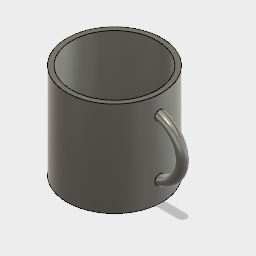
水杯 (Autodesk Fusion 360 design; units mm, degrees)
Autodesk Fusion 360 part; units mm, degrees
cylinder "圆柱体基本要素2" add diameter 20 height 20 placed x (1, 0, 0) y (0, 0, -1) z (0, 1, 0) at (0, 0, 0) makes body 1
cylinder "圆柱体基本要素3" add diameter 18 height 20 placed x (1, 0, 0) y (0, 0, -1) z (0, 1, 0) at (30, 0, 0) separate body makes body 2
torus "圆环体基本要素1" add centre line diameter 12 section diameter 2 placed x (1, 0, 0) y (0, 0, -1) z (0, 1, 0) at (65, 0, 0) separate body makes body 3
move_body "MoveFace1" bodies 3 to x (1, 0, 0) y (0, 0.173648, 0.984808) z (0, -0.984808, 0.173648) at (-80.5059, 25.9211, 54.5848) on bodies 3
move_body "移动1" bodies 2 to x (1, 0, 0) y (0, 1, 0) z (0, 0, 1) at (56.3634, -30.5498, -25.8135)
move_body "MoveFace2" bodies 3 to x (1, 0, 0) y (0, 1, 0) z (0, 0, 1) at (25.842, -18.251, -52.6794) on bodies 3
move_body "MoveFace3" bodies 3 to x (1, 0, 0) y (0, 1, 0) z (0, 0, 1) at (0, -1.3892, -7.8785) on bodies 3
move_body "MoveFace4" bodies 3 to x (1, 0, 0) y (0, 0.984808, 0.173648) z (0, -0.173648, 0.984808) at (-1.6387, 3.0344, 5.1882) on bodies 3
combine "合并1" operation add target body 3 tool bodies 1
move_body "移动2" bodies 2 to x (1, 0, 0) y (0, 1, 0) z (0, 0, 1) at (-20.0414, 19.9163, -2.5649)
move_body "对齐1" bodies 2 to x (1, 0, 0) y (0, 1, 0) z (0, 0, 1) at (0, 10.6336, 0)
move_body "对齐2" bodies 2 to x (1, 0, 0) y (0, 1, 0) z (0, 0, 1) at (0, 0, 0)
move_body "对齐3" bodies 3 to x (1, 0, 0) y (0, 1, 0) z (0, 0, 1) at (66.3219, 0, -28.3784)
move_face "偏移面1" offset -2 1 faces at (66.9895, 0, -29.4275) on bodies 2
combine "合并2" operation cut target body 3 tool bodies 2
sketch "草图5" plane through (0, 0, 0) normal (0, 1, 0) x (1, 0, 0)
